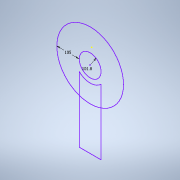
# Autodesk Inventor part: Shooter
Saved by Autodesk Inventor 2021 (Build 250183000, 183)
## iProperties
Created: 2021-04-07
Part Number: Shooter
Material: Generic
Document SubType Name: Modeling
Designer: deli
Density: 1 g/cm^3
Appearance: Default
Author: deli
Autodesk Inventor part; units mm, degrees
ref_plane "YZ Plane" through (0, 0, 0) normal (1, 0, 0) x (0, 1, 0)
ref_plane "XZ Plane" through (0, 0, 0) normal (0, 1, 0) x (-1, 0, 0)
ref_plane "XY Plane" through (0, 0, 0) normal (0, 0, 1) x (1, 0, 0)
sketch "Sketch1" plane through (0, 0, 0) normal (0, 0, 1) x (1, 0, 0)
  circle A0 centre (-7.9941, -76.1042) radius 50.9
  line L0 (42.9059, -433.1479) -> (-58.8941, -433.1479)
  arc A1 (-58.8941, -127.0042) -> (42.9059, -127.0042) centre (-7.9941, -76.1042) ccw
  line L1 (147.9059, -76.1042) -> (147.9059, -176.1042)
  line L2 (147.9059, -176.1042) -> (42.9059, -176.1042)
  line L3 (42.9059, -176.1042) -> (42.9059, -127.0042)
  line L4 (-58.8941, -176.1042) -> (-163.8941, -176.1042)
  line L5 (-163.8941, -176.1042) -> (-163.8941, -76.1042)
  line L6 (-163.8941, -76.1042) -> (-58.8941, -76.1042)
  line L7 (-58.8941, -76.1042) -> (-58.8941, -176.1042)
  line L8 (-58.8941, -176.1042) -> (42.9059, -176.1042)
  line L9 (-33.8941, -143.2668) -> (-33.8941, -176.1042)
  arc A2 (147.9059, -76.1042) -> (-163.8941, -76.1042) centre (-7.9941, -76.1042) ccw
  line L10 (-58.8941, -180.1042) -> (-167.8941, -180.1042)
  line L11 (-167.8941, -180.1042) -> (-167.8941, -76.1042)
  line L12 (-58.8941, -180.1042) -> (42.9059, -180.1042)
  line L13 (42.9059, -180.1042) -> (151.9059, -180.1042)
  line L14 (151.9059, -180.1042) -> (151.9059, -76.1042)
  arc A3 (151.9059, -76.1042) -> (-167.8941, -76.1042) centre (-7.9941, -76.1042) ccw
  line L15 (-58.8941, 79.7958) -> (-188.8941, 79.7958)
  line L16 (-188.8941, 79.7958) -> (-188.8941, -50.2042)
  line L17 (-188.8941, -50.2042) -> (-58.8941, -50.2042)
  line L18 (-58.8941, -50.2042) -> (-58.8941, 79.7958)
  line L19 (-58.8941, -76.1042) -> (-58.8941, -50.2042)
  line L20 (-58.8941, -176.1042) -> (-58.8941, -180.6362)
  line L21 (-58.8941, 79.7958) -> (-7.9941, 79.7958)
  line L22 (-188.8941, 79.7958) -> (-7.9941, 79.7958)
  line L23 (-7.9941, 79.7958) -> (-7.9941, 83.7958)
  line L24 (-7.9941, 83.7958) -> (-188.8941, 83.7958)
  line L25 (-188.8941, 83.7958) -> (-188.8941, 79.7958)
  point P0 (0, 0)
  dimension "d0" = 101.8
  dimension "d2" = 100
  dimension "d3" = 130
  dimension "d4" = 4
  dimension "d5" = 4
  dimension "d6" = 4
  dimension "d18" = 130
  dimension "d19" = 130
  constraints: 52 end point, 9 point on circle, 8 parallel, 6 perpendicular, 5 horizontal, 4 centre point, 1 coincident, 1 point on line, 1 tangent, 1 vertical, 4 other
  measures "d0" diameter of A0
  measures "d2" distance of L1.start L1.end
  measures "d3" distance between parallel lines of L5 L9
  measures "d4" distance between parallel lines of L4 L10
  measures "d5" distance between parallel lines of L8 L12
  measures "d6" distance between parallel lines of L2 L13
  measures "d18" distance of L17.end L16.end
  measures "d19" distance of L16.end L15.end
extrude "Extrusion4" add sketch "Sketch1" along normal blind 4 contours A0 | L19 L18 A2 L1 L2 L3 A1 L7 | A1 L9 L8 L7 | L17 A2 L18 | L17 A3 L18 A2 | A1 L3 L8 L9 | L8 L2 L1 A2 L23 A3 L14 L13 L12 L20 | L18 A3 L21 A2 | L17 L16 L15 L18 A3 | L21 A3 L23 | L18 L21 A3 | L21 L15 L25 L24 A3
equation "\"d20\" = d5"
body "Solid2"
